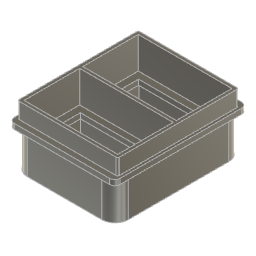
AG AA Recess v9 (Autodesk Fusion 360 design; units mm, degrees)
Autodesk Fusion 360 part; units mm, degrees
sketch "Sketch1" plane through (0, 0, 0) normal (0, 0, 1) x (1, 0, 0)
  line L0 (9.55, 12) -> (-9.55, 12)
  line L1 (-9.55, 12) -> (-9.55, -12)
  line L2 (-9.55, -12) -> (9.55, -12)
  line L3 (9.55, -12) -> (9.55, 12)
  line L4 (9.55, 12) -> (-9.55, -12) construction
  line L5 (-9.55, 12) -> (9.55, -12) construction
  line L6 (11, -13.5) -> (-11, -13.5)
  line L7 (-11, -13.5) -> (-11, 13.5)
  line L8 (-11, 13.5) -> (11, 13.5)
  line L9 (11, 13.5) -> (11, -13.5)
  line L10 (11, -13.5) -> (-11, 13.5) construction
  line L11 (-11, -13.5) -> (11, 13.5) construction
  line L12 (8.4, -10.5) -> (-8.4, -10.5)
  line L13 (-8.4, -10.5) -> (-8.4, 10.5)
  line L14 (-8.4, 10.5) -> (8.4, 10.5)
  line L15 (8.4, 10.5) -> (8.4, -10.5)
  line L16 (8.4, -10.5) -> (-8.4, 10.5) construction
  line L17 (-8.4, -10.5) -> (8.4, 10.5) construction
  line L18 (8, -9.5) -> (-8, -9.5)
  line L19 (-8, -9.5) -> (-8, 9.5)
  line L20 (-8, 9.5) -> (8, 9.5)
  line L21 (8, 9.5) -> (8, -9.5)
  line L22 (8, -9.5) -> (-8, 9.5) construction
  line L23 (-8, -9.5) -> (8, 9.5) construction
  line L24 (8.9, -0.6) -> (-8.9, -0.6)
  line L25 (-8.9, -0.6) -> (-8.9, 0.6)
  line L26 (-8.9, 0.6) -> (8.9, 0.6)
  line L27 (8.9, 0.6) -> (8.9, -0.6)
  line L28 (8.9, -0.6) -> (-8.9, 0.6) construction
  line L29 (-8.9, -0.6) -> (8.9, 0.6) construction
  line L30 (9.55, -1.5) -> (-9.55, -1.5)
  line L31 (-9.55, -1.5) -> (-9.55, 1.5)
  line L32 (-9.55, 1.5) -> (9.55, 1.5)
  line L33 (9.55, 1.5) -> (9.55, -1.5)
  line L34 (9.55, -1.5) -> (-9.55, 1.5) construction
  line L35 (-9.55, -1.5) -> (9.55, 1.5) construction
  dimension "d1" = 19.1
  dimension "d2" = 24
  dimension "d3" = 22
  dimension "d4" = 27
  dimension "d5" = 16.8
  dimension "d6" = 21
  dimension "d7" = 16
  dimension "d8" = 19
  dimension "d27" = 1.2
  dimension "d36" = 3
  constraint horizontal L0
  constraint perpendicular L0 L1
  constraint parallel L0 L2
  constraint parallel L1 L3
  constraint coincident L4 origin
  constraint coincident L5 origin
  constraint horizontal L6
  constraint perpendicular L6 L7
  constraint parallel L6 L8
  constraint parallel L7 L9
  constraint coincident L10 origin
  constraint coincident L11 origin
  constraint horizontal L12
  constraint perpendicular L12 L13
  constraint parallel L12 L14
  constraint parallel L13 L15
  constraint coincident L16 origin
  constraint coincident L17 origin
  constraint horizontal L18
  constraint perpendicular L18 L19
  constraint parallel L18 L20
  constraint parallel L19 L21
  constraint coincident L22 origin
  constraint coincident L23 origin
  constraint horizontal L24
  constraint perpendicular L24 L25
  constraint parallel L24 L26
  constraint parallel L25 L27
  constraint coincident L28 origin
  constraint coincident L29 origin
  constraint horizontal L30
  constraint perpendicular L30 L31
  constraint parallel L30 L32
  constraint parallel L31 L33
  constraint coincident L34 origin
  constraint coincident L35 origin
  measures "d1" distance of L1.end L2.end
  measures "d2" distance of L0.end L1.end
  measures "d3" distance of L7.end L8.end
  measures "d4" distance of L6.end L7.end
  measures "d5" distance of L13.end L14.end
  measures "d6" distance of L12.end L13.end
  measures "d7" distance of L19.end L20.end
  measures "d8" distance of L18.end L19.end
  measures "d27" distance of L24.end L25.end
  measures "d36" distance of L30.end L31.end
extrude "Extrude1" add sketch "Sketch1" along normal blind 1 contours L13 L14 L15 L19 L20 L21 L32 | L15 L21 L26 L32 | L13 L19 L26 L32 | L15 L21 L24 L30 | L12 L13 L15 L18 L19 L21 L30 | L15 L21 L24 L26 | L13 L19 L24 L30 | L13 L19 L24 L26
extrude "Extrude2" add sketch "Sketch1" along normal blind 7 contours L0 L1 L3 L13 L14 L15 L32 | L3 L15 L24 L26 L27 L30 L32 L33 | L1 L13 L24 L25 L26 L30 L31 L32 | L1 L2 L3 L12 L13 L15 L30 | L15 L24 L26 L27 | L13 L24 L25 L26
extrude "Extrude3" add sketch "Sketch1" along normal blind 8
extrude "Extrude4" cut sketch "Sketch1" along normal blind 7
extrude "Extrude5" add 1 faces at (2.8, -11.5, 7) along direction (0, 0, 1) blind 1
extrude "Extrude6" add sketch "Sketch1" along normal blind 8 contours L15 L21 L24 L26 | L13 L19 L24 L26 | L19 L21 L24 L26
fillet "Fillet6" radius 2.5 4 edges at (9.55, 12, 3.5) (9.55, -12, 3.5) (-9.55, 12, 3.5) (-9.55, -12, 3.5)
fillet "Fillet7" radius 1 4 edges at (11, -13.5, 7.5) (-11, -13.5, 7.5) (11, 13.5, 7.5) (-11, 13.5, 7.5)
extrude "Extrude7" add sketch "Sketch1" along normal blind 1 contours L3 L15 L24 L26 L27 L30 L32 L33 | L1 L13 L24 L25 L26 L30 L31 L32 | L15 L21 L26 L32 | L13 L19 L26 L32 | L15 L21 L24 L30 | L19 L21 L26 L32 | L13 L19 L24 L30 | L19 L21 L24 L30
extrude "Extrude8" add 2 faces at (2.6667, -10.1667, 1) (2.6667, 10.1667, 1) along direction (0, 0, 1) blind 5
extrude "Extrude9" cut sketch "Sketch1" along normal blind 4 contours L13 L14 L15 L19 L20 L21 L32 | L15 L21 L26 L32 | L13 L19 L26 L32 | L15 L21 L24 L30 | L12 L13 L15 L18 L19 L21 L30 | L19 L21 L26 L32 | L13 L19 L24 L30 | L19 L21 L24 L30
extrude "Extrude10" add 2 faces at (-8, -6.8333, 4.6667) (-8, 4.1667, 4.6667) along direction (1, 0, 0) blind 0.5
extrude "Extrude11" add 2 faces at (8, 6.8333, 4.6667) (8, -4.1667, 5.3333) along direction (-1, 0, 0) blind 0.5
extrude "Extrude12" cut 2 faces at (-8.4, -3.9, 6.6667) (-8.4, 7.2, 6.6667) along direction (-1, 0, 0) blind 0.15
extrude "Extrude13" cut 2 faces at (8.4, 3.9, 6.6667) (8.4, -7.2, 6.6667) along direction (1, 0, 0) blind 0.15
extrude "Extrude14" cut 1 faces at (2.85, 10.5, 6.6667) along direction (0, 1, 0) blind 0.3
extrude "Extrude15" cut 1 faces at (2.85, -0.6, 7.3333) along direction (0, 1, 0) blind 0.3
extrude "Extrude16" cut 2 faces at (8.55, 4, 6.6667) (8.55, -7.1, 7.3333) along direction (1, 0, 0) blind 0.3
extrude "Extrude17" cut 2 faces at (-8.55, -3.7, 6.6667) (-8.55, 7.4, 6.6667) along direction (-1, 0, 0) blind 0.3
extrude "Extrude18" cut 1 faces at (-2.95, 0.6, 7.3333) along direction (0, -1, 0) blind 0.3
extrude "Extrude19" cut 1 faces at (-2.95, -10.5, 7.3333) along direction (0, -1, 0) blind 0.3
extrude "Extrude20" cut 2 faces at (8.4, -6.8667, 6) (8.4, 6.8667, 6) along direction (0, 0, -1) blind 1
extrude "Extrude21" add 1 faces at (-2.95, 12.6, 8) along direction (0, 0, 1) blind 3
sketch "Sketch2" plane through (0, 0, 11) normal (0, 0, 1) x (-1, 0, 0)
  arc A0 (10, -13.5) -> (11, -12.5) centre (10, -12.5) ccw
  line L0 (11, -12.5) -> (11, 12.5)
  arc A1 (11, 12.5) -> (10, 13.5) centre (10, 12.5) ccw
  line L1 (10, 13.5) -> (-10, 13.5)
  arc A2 (-10, 13.5) -> (-11, 12.5) centre (-10, 12.5) ccw
  line L2 (-11, 12.5) -> (-11, -12.5)
  arc A3 (-11, -12.5) -> (-10, -13.5) centre (-10, -12.5) ccw
  line L3 (-10, -13.5) -> (10, -13.5)
  line L4 (-8.85, -10.8) -> (-8.85, -0.3)
  line L5 (-8.85, -0.3) -> (8.85, -0.3)
  line L6 (8.85, -0.3) -> (8.85, -10.8)
  line L7 (8.85, -10.8) -> (-8.85, -10.8)
  line L8 (-8.85, 0.3) -> (-8.85, 10.8)
  line L9 (-8.85, 10.8) -> (8.85, 10.8)
  line L10 (8.85, 10.8) -> (8.85, 0.3)
  line L11 (8.85, 0.3) -> (-8.85, 0.3)
  line L12 (-9.463, 11.4127) -> (9.463, 11.4127)
  line L13 (9.463, 11.4127) -> (9.463, -11.4127)
  line L14 (9.463, -11.4127) -> (-9.463, -11.4127)
  line L15 (-9.463, -11.4127) -> (-9.463, 11.4127)
  line L16 (-9.463, 11.4127) -> (9.463, -11.4127) construction
  line L17 (9.463, 11.4127) -> (-9.463, -11.4127) construction
  constraint horizontal L12
  constraint perpendicular L12 L13
  constraint parallel L12 L14
  constraint parallel L13 L15
  constraint coincident L16 origin
  constraint coincident L17 origin
extrude "Extrude22" cut sketch "Sketch2" against normal blind 3 contours A0 L0 A1 L1 A2 L2 A3 L3
fillet "Fillet8" radius 0.3 4 edges at (9.463, -11.4127, 9.5) (-9.463, -11.4127, 9.5) (-9.463, 11.4127, 9.5) (9.463, 11.4127, 9.5)
delete_face "DeleteFace1" 1 faces at (-10.4582, 13.3888, 7.3333)
delete_face "DeleteFace2" 1 faces at (-10.2358, -13.4718, 7.6667)
delete_face "DeleteFace3" 1 faces at (10.9955, -12.5951, 7.3333)
delete_face "DeleteFace4" 1 faces at (10.0476, 13.4989, 7.6667)
extrude "Extrude25" cut 1 faces at (3.6667, -13.5, 7.6667) along direction (0, 1, 0) blind 1
extrude "Extrude26" cut 1 faces at (-3.6667, 13.5, 7.6667) along direction (0, -1, 0) blind 1
extrude "Extrude27" cut 1 faces at (-11, -4.1667, 7.3333) along direction (1, 0, 0) blind 1
extrude "Extrude28" cut 1 faces at (11, 4.1667, 7.3333) along direction (-1, 0, 0) blind 1
fillet "Fillet9" radius 1 4 edges at (10, -12.5, 7.5) (-10, -12.5, 7.5) (-10, 12.5, 7.5) (10, 12.5, 7.5)
extrude "Extrude23" [suppressed]
extrude "Extrude24" [suppressed]
